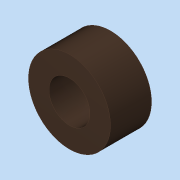
# Autodesk Inventor part: SleeveBearing.125inch
Saved by Autodesk Inventor 2017 (Build 210142000, 142)
## iProperties
Created: 2016-11-06
Part Number: SleeveBearing.125inch
Material: Bronze, Cast
Document SubType Name: Modeling
Designer: techn
Density: 8.87 g/cm^3
Appearance: Bronze - Satin
Author: techn
Autodesk Inventor part; units mm, degrees
ref_plane "YZ Plane" through (0, 0, 0) normal (1, 0, 0) x (0, 1, 0)
ref_plane "XZ Plane" through (0, 0, 0) normal (0, 1, 0) x (-1, 0, 0)
ref_plane "XY Plane" through (0, 0, 0) normal (0, 0, 1) x (1, 0, 0)
sketch "Sketch1" plane through (0, 0, 0) normal (0, 0, 1) x (1, 0, 0)
  circle A0 centre (0, 0) radius 1.5875
  circle A1 centre (0, 0) radius 3.175
  dimension "d0" = 3.175
  dimension "d1" = 6.35
  constraints: 2 centre point, 2 coincident
  measures "d0" diameter of A0
  measures "d1" diameter of A1
extrude "Extrusion1" add sketch "Sketch1" along normal blind 3.175
body "Solid1"
